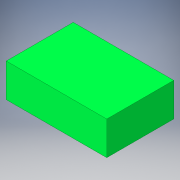
# Autodesk Inventor part: 3 x2
Saved by Autodesk Inventor 2016 (Build 200138000, 138)
## iProperties
Created: 2016-07-21
Part Number: 3 x2
Material: Generic
Document SubType Name: Modeling
Designer: cfkguest
Density: 1 g/cm^3
Appearance: Default
Author: cfkguest
Autodesk Inventor part; units mm, degrees
ref_plane "YZ Plane" through (0, 0, 0) normal (1, 0, 0) x (0, 1, 0)
ref_plane "XZ Plane" through (0, 0, 0) normal (0, 1, 0) x (-1, 0, 0)
ref_plane "XY Plane" through (0, 0, 0) normal (0, 0, 1) x (1, 0, 0)
sketch "Sketch1" plane through (0, 0, 0) normal (0, 0, 1) x (1, 0, 0)
  line L0 (-19.2482, 19.3849) -> (56.9518, 19.3849)
  line L1 (56.9518, 19.3849) -> (56.9518, -6.0151)
  line L2 (56.9518, -6.0151) -> (-19.2482, -6.0151)
  line L3 (-19.2482, -6.0151) -> (-19.2482, 19.3849)
  point P0 (0, 0)
  dimension "d0" = 76.2
  dimension "d1" = 25.4
  constraints: 8 end point, 2 parallel, 1 horizontal, 1 perpendicular
  measures "d0" distance of L1.end L2.end
  measures "d1" distance of L2.end L0.start
extrude "Extrusion1" add sketch "Sketch1" along normal blind 50.8
body "Solid1"
